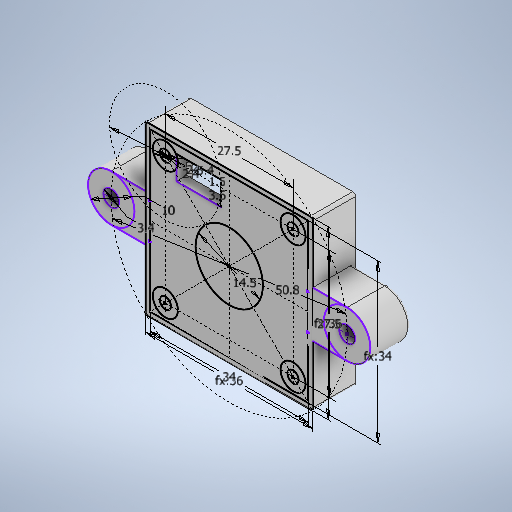
# Autodesk Inventor part: cameraBottom
Saved by Autodesk Inventor 2025 (Build 290162000, 162)
## iProperties
Created: 2025-03-10
Part Number: cameraBottom
Material: Generic
Document SubType Name: Modeling
Designer: john
Density: 1 g/cm^3
Appearance: Default
Author: john
Autodesk Inventor part; units mm, degrees
ref_plane "YZ Plane" through (0, 0, 0) normal (1, 0, 0) x (0, 1, 0)
ref_plane "XZ Plane" through (0, 0, 0) normal (0, 1, 0) x (-1, 0, 0)
ref_plane "XY Plane" through (0, 0, 0) normal (0, 0, 1) x (1, 0, 0)
sketch "Sketch1" plane through (0, 0, 0) normal (0, 0, 1) x (1, 0, 0)
  circle A0 centre (0, 0) radius 25.4 construction
  line L0 (-13.75, -13.75) -> (13.75, -13.75) construction
  line L1 (13.75, -13.75) -> (13.75, 13.75) construction
  line L2 (13.75, 13.75) -> (-13.75, 13.75) construction
  line L3 (-13.75, 13.75) -> (-13.75, -13.75) construction
  line L4 (-13.75, -13.75) -> (13.75, 13.75) construction
  line L5 (13.75, -13.75) -> (-13.75, 13.75) construction
  circle A1 centre (0, 0) radius 7.25
  circle A2 centre (-13.75, 13.75) radius 1.2
  circle A3 centre (-13.75, 13.75) radius 2.7
  circle A4 centre (-25.4, 0) radius 1.7
  circle A5 centre (-25.4, 0) radius 5
  line L6 (-17, 17) -> (17, 17)
  line L7 (17, 17) -> (17, -17)
  line L8 (17, -17) -> (-17, -17)
  line L9 (-17, -17) -> (-17, 17)
  line L10 (-17, 17) -> (17, -17) construction
  line L11 (17, 17) -> (-17, -17) construction
  line L12 (-25.4, 5) -> (-18, 5)
  line L13 (-25.4, -5) -> (-18, -5)
  line L14 (0, 17) -> (0, -17) construction
  line L15 (-17, 0) -> (17, 0) construction
  circle A6 centre (25.4, 0) radius 1.7
  circle A7 centre (25.4, 0) radius 5
  line L16 (25.4, 5) -> (18, 5)
  line L17 (25.4, -5) -> (18, -5)
  circle A8 centre (13.75, 13.75) radius 1.2
  circle A9 centre (13.75, 13.75) radius 2.7
  circle A10 centre (-13.75, -13.75) radius 1.2
  circle A11 centre (-13.75, -13.75) radius 2.7
  circle A12 centre (13.75, -13.75) radius 2.7
  circle A13 centre (13.75, -13.75) radius 1.2
  line L18 (-18, 18) -> (18, 18)
  line L19 (18, 18) -> (18, -18)
  line L20 (18, -18) -> (-18, -18)
  line L21 (-18, -18) -> (-18, 18)
  line L22 (-18, 18) -> (18, -18) construction
  line L23 (18, 18) -> (-18, -18) construction
  circle A14 centre (-13.75, 13.75) radius 12 construction
  line L24 (-1.75, 13.75) -> (-1.75, 15.25) construction
  line L25 (-1.75, 13.75) -> (-1.75, 10.15) construction
  line L26 (-11.35, 13.75) -> (-11.35, 10.15) construction
  line L27 (-11.35, 13.75) -> (-11.35, 15.25) construction
  line L28 (-11.35, 10.15) -> (-1.75, 10.15)
  line L29 (-1.75, 10.15) -> (-1.75, 15.25)
  line L30 (-1.75, 15.25) -> (-11.35, 15.25)
  line L31 (-11.35, 15.25) -> (-11.35, 10.15)
  point P0 (-17, 3.8)
  point P1 (-17, -3.8)
  point P2 (17, 3.8)
  point P3 (17, -3.8)
  dimension "d22" = 24
  dimension "d0" = 50.8
  dimension "d1" = 27.5
  dimension "d2" = 27.5
  dimension "d3" = 14.5
  dimension "d4" = 2.4
  dimension "d5" = 5.4
  dimension "d6" = 3.4
  dimension "d7" = 10
  dimension "d8" = 34
  dimension "d9" = 34
  dimension "d10" = 36
  dimension "d11" = 36
  dimension "d24" = 1.5
  dimension "d25" = 3.6
  constraints: 64 end point, 18 coincident, 14 centre point, 12 symmetric about line, 10 midpoint, 9 point on line, 8 parallel, 7 perpendicular, 6 point on circle, 4 horizontal, 4 vertical, 2 tangent, 1 horizontal alignment, 10 other
  measures "d0" diameter of A0
  measures "d1" distance of L2.end L1.end
  measures "d2" distance of L1.end L0.end
  measures "d3" diameter of A1
  measures "d4" diameter of A2
  measures "d5" diameter of A3
  measures "d6" diameter of A4
  measures "d7" diameter of A5
  measures "d8" distance of L7.end L8.end
  measures "d9" distance of L6.end L7.end
  measures "d10" distance of L19.end L20.end
  measures "d11" distance of L18.end L19.end
  measures "d24" distance of L24.start L24.end
  measures "d25" distance of L24.start L25.end
extrude "Extrusion1" add sketch "Sketch1" against normal blind 9.2 contours L21 L18 L19 L20
extrude "Extrusion3" add sketch "Sketch1" against normal blind 7.4 contours A3 L31 | L31 A3 | A9 | A11 | A12
extrude "Extrusion4" add sketch "Sketch1" against normal blind 2.2 contours A1 | A2 | A3 L31 L30 L29 L28 | L6 L7 L8 L9 | A8 | A10 | A13
extrude "Extrusion5" add sketch "Sketch1" against normal blind 8.65 contours A5 | A5 L12 L21 L13 | L16 A7 L17 L19 | A7
extrude "Extrusion6" cut sketch "Sketch1" along normal mid plane 22 contours A3 L31 | A3 L31 L30 L29 L28 picked at (-11.2949, 13.4692)
fillet "Fillet1" radius 0.6 10 edges at (-18, -18, -4.6) (-18, 18, -4.6) (18, 18, -4.6) (18, -18, -4.6) (-30.4, 0, -8.65) (-21.7, 5, -8.65) (-21.7, -5, -8.65) (30.4, 0, -8.65) (21.7, 5, -8.65) (21.7, -5, -8.65)
equation "\"d9\" = d8"
body "Solid1"
